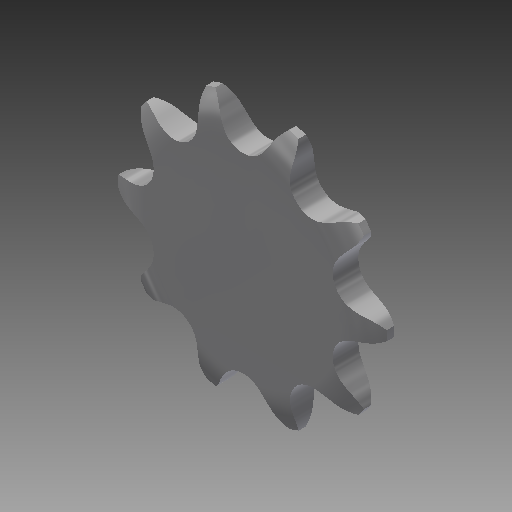
# Autodesk Inventor part: Roller Chain Sprocket2
Saved by Autodesk Inventor 2019.4 (Build 234330000, 330)
## iProperties
Created: 2020-01-11
Part Number: Roller Chain Sprocket2
Material: Steel
Document SubType Name: Modeling
Designer: admin
Density: 1 g/cm^3
Appearance: Steel
CustomPartVersion: 1
Author: admin
Autodesk Inventor part; units mm, degrees
ref_plane "YZ Plane" through (0, 0, 0) normal (1, 0, 0) x (0, 1, 0)
ref_plane "XZ Plane" through (0, 0, 0) normal (0, 1, 0) x (-1, 0, 0)
ref_plane "XY Plane" through (0, 0, 0) normal (0, 0, 1) x (1, 0, 0)
sketch "Theoretical Tooth Profile" plane through (0, 0, 0) normal (0, 0, 1) x (1, 0, 0)
  circle A0 centre (0, 0) radius 12.9443 construction
  line L0 (0, 0) -> (0, 12.9443) construction
  line L1 (0, 0) -> (7.6085, 10.4721) construction
  circle A1 centre (0, 0) radius 14.7107
  arc A2 (-1.9056, 11.2877) -> (1.9056, 11.2877) centre (0, 12.9443) ccw
  line L2 (0, 12.9443) -> (7.6085, 10.4721) construction
  line L3 (0, 12.9443) -> (3.0188, 15.5685) construction
  line L4 (3.0188, 15.5685) -> (-2.71, 12.445) construction
  arc A3 (4.04, 14.1451) -> (2.9152, 12.8215) centre (6.6574, 10.7812) ccw
  arc A4 (-2.9152, 12.8215) -> (-4.04, 14.1451) centre (-6.6574, 10.7812) ccw
  line L5 (-6.6574, 10.7812) -> (-2.9152, 12.8215) construction
  arc A5 (-2.71, 12.445) -> (-1.9056, 11.2877) centre (3.0188, 15.5685) ccw
  line L6 (-2.71, 12.445) -> (-2.9152, 12.8215)
  arc A6 (1.9056, 11.2877) -> (2.71, 12.445) centre (-3.0188, 15.5685) ccw
  line L7 (2.9152, 12.8215) -> (2.71, 12.445)
  line L8 (0, 0) -> (4.5459, 13.9907) construction
  point P0 (3.8042, 11.7082)
  dimension "d0" = 25.8885
  dimension "d2" = 36
  dimension "d3" = 2.525
  dimension "d10" = 131
  dimension "d11" = 12.4
  dimension "d12" = 4
  dimension "d13" = 6.525
  dimension "d14" = 7
  dimension "d23" = 2.4
  constraints: 18 end point, 15 point on circle, 7 centre point, 3 coincident, 3 point on line, 3 symmetric about line, 3 tangent, 1 equal radius, 1 midpoint, 1 parallel, 1 vertical, 1 other
  measures "d0" diameter of A0
  measures "d2" angle of L1 L0
  measures "d3" radius of A2
  measures "d10" angle of L3 L0
  measures "d11" angle of L4 L3
  measures "d12" distance of L2.start L3.end
  measures "d13" distance of L3.end L4.end
  measures "d14" distance of A3.centre L0.end
  measures "d23" distance from line of L8.end L2
sketch "Tooth Profile" plane through (0, 0, 0) normal (0, 0, 1) x (1, 0, 0)
  arc A0 (-2.2977, 11.8972) -> (2.2977, 11.8972) centre (0, 12.9443) ccw
  arc A1 (3.936, 14.1744) -> (2.2977, 11.8972) centre (8.8494, 8.9114) ccw
  arc A2 (-2.2977, 11.8972) -> (-3.936, 14.1744) centre (-8.8494, 8.9114) ccw
  line L0 (0, 0) -> (0, 12.9443) construction
  line L1 (0, 12.9443) -> (2.2977, 11.8972) construction
  line L2 (0, 12.9443) -> (-2.2977, 11.8972) construction
  circle A3 centre (0, 0) radius 14.7107 projected
  dimension "d44" = 131
  dimension "d45" = 7.2
  dimension "d46" = 2.525
  constraints: 9 point on circle, 6 end point, 3 centre point, 2 tangent, 1 coincident, 1 equal radius, 1 vertical, 1 other
  measures "d44" angle of L2 L1
  measures "d45" radius of A1
  measures "d46" radius of A0
sketch "Section Profile" plane through (0, 0, 0) normal (1, 0, 0) x (0, 1, 0)
  line L0 (14.7107, 0) -> (-14.7107, 0) projected
  line L1 (4.4935, 1.395) -> (-4.4935, 1.395)
  line L2 (-4.4935, 1.395) -> (-4.4935, -1.395)
  line L3 (-4.4935, -1.395) -> (4.4935, -1.395)
  line L4 (4.4935, -1.395) -> (4.4935, 1.395)
  line L5 (4.4935, 1.395) -> (14.7107, 1.395) construction
  line L6 (14.7107, 1.395) -> (14.7107, -1.395) construction
  line L7 (14.7107, -1.395) -> (4.4935, -1.395) construction
  line L8 (4.4935, -1.395) -> (4.4935, 1.395)
  arc A0 (14.7107, 0.395) -> (10.8378, 1.395) centre (10.8378, -6.605) ccw
  arc A1 (10.8378, -1.395) -> (14.7107, -0.395) centre (10.8378, 6.605) ccw
  line L9 (10.8378, 1.395) -> (0, 1.395)
  line L10 (0, 1.395) -> (0, -1.395)
  line L11 (0, -1.395) -> (10.8378, -1.395)
  line L12 (0, 1.395) -> (0, -1.395)
  line L13 (14.7107, 0.395) -> (14.7107, -0.395)
  point P0 (0, 0)
  point P1 (0, 0)
  dimension "d30" = 2.79
  dimension "d31" = 8.9871
  dimension "d32" = 2.79
  dimension "d33" = 1
  dimension "d34" = 8
  dimension "d43" = 1.395
  constraints: 26 end point, 7 midpoint, 5 perpendicular, 4 parallel, 4 point on circle, 3 point on line, 3 symmetric about line, 2 centre point, 2 horizontal, 2 tangent, 1 collinear, 1 other
  measures "d30" distance between parallel lines of L7 L5
  measures "d31" distance between parallel lines of L2 L4
  measures "d32" distance between parallel lines of L3 L1
  measures "d33" distance from line of L13.start L5
  measures "d34" radius of A0
  measures "d43" distance between parallel lines of L3 L0
revolve "Shroud" add sketch "Section Profile" angle 360 about axis through (0, 0, 1.395) along (0, 0, -1) contours L10 L3 L2 L0 | L0 L2 L1 L10
revolve "Strand" add sketch "Section Profile" angle 360 about axis through (0, 0, 1.395) along (0, 0, -1) contours L13 A1 L11 L4 L0 | L0 L4 L9 A0 L13 | L4 L3 L10 L0 | L0 L10 L1 L4
pattern_of_one "Strand Pattern"
extrude "Theoretical Tooth" cut sketch "Theoretical Tooth Profile" along normal through all both and the other way through all contours A3 L7 A6 A2 A5 L6 A4 A1 picked at (0.1026, 13.2444)
extrude "Tooth" [suppressed]
pattern_circular "Tooth Pattern" count 10 over 360 about axis through (0, 0, -10) along (0, 0, 1) of "Theoretical Tooth"
ref_plane "Timing Plane" through (0, 12.9443, 0) normal (1, 0, 0) x (0, 1, 0)
equation "\"d3\" = 0.5 * da_Dr + da_SC"
equation "\"d12\" = 0.8 * da_Dr"
equation "\"d13\" = 1.3 * da_Dr + da_SC"
equation "\"d14\" = 1.4 * da_Dr"
equation "\"d23\" = da_Ha"
equation "\"d44\" = da_Alfa"
equation "\"d45\" = da_Re"
equation "\"d46\" = da_Ri"
equation "\"d30\" = da_Bf"
equation "\"d31\" = da_Ds"
equation "\"d32\" = da_Bs"
equation "\"d33\" = da_Ba"
equation "\"d34\" = da_Rx"
equation "\"d40\" = da_pt"
equation "\"form_type\" = 0"
equation "\"da_p\" = 8"
equation "\"da_Dr\" = 5"
equation "\"da_SC\" = 0.025"
equation "\"da_Ha\" = 2.4"
equation "\"da_pt\" = 5.64"
equation "\"da_Bf\" = 2.79"
equation "\"da_Ba\" = 1"
equation "\"da_Rx\" = 8"
equation "\"da_Ra\" = 0.32"
equation "\"da_Bs\" = 2.79"
equation "\"da_Ds\" = 8.98707"
equation "\"da_Re\" = 7.2"
equation "\"da_Ri\" = 2.525"
equation "\"da_Alfa\" = 131deg"
body "Solid1"
